Autodesk Fusion 360 part; units mm, degrees
note: some values were not read from the file. Chosen so that the rebuilt part matches the saved one: which bodies a step acts on.
(part 2 of 3)
  line L404 (275.1852, -92.964) -> (274.8216, -92.964)
  line L405 (274.8216, -92.964) -> (274.8216, -90.0604)
  arc A366 (268.6669, -89.5604) -> (268.1669, -90.0604) centre (268.6669, -90.0604) ccw
  arc A367 (268.1669, -101.5666) -> (267.6669, -101.0666) centre (267.6669, -101.5666) ccw
  arc A368 (269.9703, -102.354) -> (269.4703, -101.854) centre (269.4703, -102.354) ccw
  arc A369 (269.9703, -102.5224) -> (270.4703, -103.0224) centre (270.4703, -102.5224) ccw
  arc A370 (272.5183, -103.0224) -> (273.0183, -102.5224) centre (272.5183, -102.5224) ccw
  arc A371 (273.5183, -101.854) -> (273.0183, -102.354) centre (273.5183, -102.354) ccw
  arc A372 (274.3216, -101.854) -> (274.8216, -101.354) centre (274.3216, -101.354) ccw
  arc A373 (275.3216, -95.758) -> (274.8216, -96.258) centre (275.3216, -96.258) ccw
  arc A374 (275.6852, -93.464) -> (275.1852, -92.964) centre (275.1852, -93.464) ccw
  arc A375 (274.8216, -90.0604) -> (274.3216, -89.5604) centre (274.3216, -90.0604) ccw
  line L406 (293.5375, -88.25) -> (306.5375, -88.25)
  line L407 (293.5375, -102.25) -> (306.5375, -102.25)
  line L408 (293.0375, -88.75) -> (293.0375, -101.75)
  line L409 (307.0375, -88.75) -> (307.0375, -101.75)
  arc A376 (293.5375, -88.25) -> (293.0375, -88.75) centre (293.5375, -88.75) ccw
  arc A377 (307.0375, -88.75) -> (306.5375, -88.25) centre (306.5375, -88.75) ccw
  arc A378 (293.0375, -101.75) -> (293.5375, -102.25) centre (293.5375, -101.75) ccw
  arc A379 (306.5375, -102.25) -> (307.0375, -101.75) centre (306.5375, -101.75) ccw
  line L410 (312.5875, -88.25) -> (325.5875, -88.25)
  line L411 (312.5875, -102.25) -> (325.5875, -102.25)
  line L412 (312.0875, -88.75) -> (312.0875, -101.75)
  line L413 (326.0875, -88.75) -> (326.0875, -101.75)
  arc A380 (312.5875, -88.25) -> (312.0875, -88.75) centre (312.5875, -88.75) ccw
  arc A381 (326.0875, -88.75) -> (325.5875, -88.25) centre (325.5875, -88.75) ccw
  arc A382 (312.0875, -101.75) -> (312.5875, -102.25) centre (312.5875, -101.75) ccw
  arc A383 (325.5875, -102.25) -> (326.0875, -101.75) centre (325.5875, -101.75) ccw
  line L414 (331.6375, -88.25) -> (344.6375, -88.25)
  line L415 (331.6375, -102.25) -> (344.6375, -102.25)
  line L416 (331.1375, -88.75) -> (331.1375, -101.75)
  line L417 (345.1375, -88.75) -> (345.1375, -101.75)
  arc A384 (331.6375, -88.25) -> (331.1375, -88.75) centre (331.6375, -88.75) ccw
  arc A385 (345.1375, -88.75) -> (344.6375, -88.25) centre (344.6375, -88.75) ccw
  arc A386 (331.1375, -101.75) -> (331.6375, -102.25) centre (331.6375, -101.75) ccw
  arc A387 (344.6375, -102.25) -> (345.1375, -101.75) centre (344.6375, -101.75) ccw
  line L418 (5.4062, -107.3) -> (18.4063, -107.3)
  line L419 (5.4062, -121.3) -> (18.4063, -121.3)
  line L420 (4.9062, -107.8) -> (4.9062, -120.8)
  line L421 (18.9062, -107.8) -> (18.9062, -120.8)
  arc A388 (5.4062, -107.3) -> (4.9062, -107.8) centre (5.4062, -107.8) ccw
  arc A389 (18.9062, -107.8) -> (18.4062, -107.3) centre (18.4062, -107.8) ccw
  arc A390 (4.9062, -120.8) -> (5.4062, -121.3) centre (5.4062, -120.8) ccw
  arc A391 (18.4062, -121.3) -> (18.9063, -120.8) centre (18.4062, -120.8) ccw
  line L422 (29.2188, -107.3) -> (42.2188, -107.3)
  line L423 (29.2188, -121.3) -> (42.2188, -121.3)
  line L424 (28.7188, -107.8) -> (28.7188, -120.8)
  line L425 (42.7188, -107.8) -> (42.7188, -120.8)
  arc A392 (29.2188, -107.3) -> (28.7187, -107.8) centre (29.2188, -107.8) ccw
  arc A393 (42.7188, -107.8) -> (42.2188, -107.3) centre (42.2188, -107.8) ccw
  arc A394 (28.7188, -120.8) -> (29.2188, -121.3) centre (29.2188, -120.8) ccw
  arc A395 (42.2188, -121.3) -> (42.7188, -120.8) centre (42.2188, -120.8) ccw
  line L426 (53.0313, -107.3) -> (66.0312, -107.3)
  line L427 (53.0313, -121.3) -> (66.0312, -121.3)
  line L428 (52.5313, -107.8) -> (52.5313, -120.8)
  line L429 (66.5312, -107.8) -> (66.5312, -120.8)
  arc A396 (53.0313, -107.3) -> (52.5312, -107.8) centre (53.0313, -107.8) ccw
  arc A397 (66.5312, -107.8) -> (66.0312, -107.3) centre (66.0312, -107.8) ccw
  arc A398 (52.5313, -120.8) -> (53.0313, -121.3) centre (53.0313, -120.8) ccw
  arc A399 (66.0312, -121.3) -> (66.5312, -120.8) centre (66.0312, -120.8) ccw
  line L430 (124.4688, -107.3) -> (137.4688, -107.3)
  line L431 (124.4688, -121.3) -> (137.4688, -121.3)
  line L432 (123.9688, -107.8) -> (123.9688, -120.8)
  line L433 (137.9688, -107.8) -> (137.9688, -120.8)
  arc A400 (124.4688, -107.3) -> (123.9688, -107.8) centre (124.4688, -107.8) ccw
  arc A401 (137.9688, -107.8) -> (137.4688, -107.3) centre (137.4688, -107.8) ccw
  arc A402 (123.9688, -120.8) -> (124.4688, -121.3) centre (124.4688, -120.8) ccw
  arc A403 (137.4688, -121.3) -> (137.9688, -120.8) centre (137.4688, -120.8) ccw
  line L434 (78.1414, -108.6104) -> (83.7961, -108.6104)
  line L435 (84.2961, -109.1104) -> (84.2961, -111.5)
  line L436 (84.7962, -112) -> (130.9688, -112)
  line L437 (130.9688, -116.6) -> (84.7961, -116.6)
  line L438 (84.2961, -117.1) -> (84.2961, -120.404)
  line L439 (83.7961, -120.904) -> (82.9928, -120.904)
  line L440 (82.4928, -121.404) -> (82.4928, -121.5724)
  line L441 (81.9928, -122.0724) -> (79.9447, -122.0724)
  line L442 (79.4447, -121.5724) -> (79.4447, -121.404)
  line L443 (78.9447, -120.904) -> (78.1414, -120.904)
  line L444 (77.6414, -120.404) -> (77.6414, -115.308)
  line L445 (77.1414, -114.808) -> (76.7777, -114.808)
  line L446 (76.7777, -114.808) -> (76.7777, -112.514)
  line L447 (77.2777, -112.014) -> (77.6414, -112.014)
  line L448 (77.6414, -112.014) -> (77.6414, -109.1104)
  arc A404 (84.2962, -109.1104) -> (83.7961, -108.6104) centre (83.7961, -109.1104) ccw
  arc A405 (84.2962, -111.5) -> (84.7962, -112) centre (84.7962, -111.5) ccw
  arc A406 (84.7962, -116.6) -> (84.2962, -117.1) centre (84.7962, -117.1) ccw
  arc A407 (83.7961, -120.904) -> (84.2962, -120.404) centre (83.7961, -120.404) ccw
  arc A408 (82.9928, -120.904) -> (82.4928, -121.404) centre (82.9928, -121.404) ccw
  arc A409 (81.9928, -122.0724) -> (82.4927, -121.5724) centre (81.9928, -121.5724) ccw
  arc A410 (79.4447, -121.5724) -> (79.9447, -122.0724) centre (79.9447, -121.5724) ccw
  arc A411 (79.4447, -121.404) -> (78.9447, -120.904) centre (78.9447, -121.404) ccw
  arc A412 (77.6414, -120.404) -> (78.1414, -120.904) centre (78.1414, -120.404) ccw
  arc A413 (77.6414, -115.308) -> (77.1414, -114.808) centre (77.1414, -115.308) ccw
  arc A414 (77.2777, -112.014) -> (76.7777, -112.514) centre (77.2777, -112.514) ccw
  arc A415 (78.1414, -108.6104) -> (77.6414, -109.1104) centre (78.1414, -109.1104) ccw
  line L449 (183.7962, -108.6104) -> (178.1413, -108.6104)
  line L450 (177.6413, -109.1104) -> (177.6413, -111.5)
  line L451 (177.1413, -112) -> (130.9688, -112)
  line L452 (130.9688, -116.6) -> (177.1413, -116.6)
  line L453 (177.6413, -117.1) -> (177.6413, -120.404)
  line L454 (178.1413, -120.904) -> (178.9447, -120.904)
  line L455 (179.4447, -121.404) -> (179.4447, -121.5724)
  line L456 (179.9447, -122.0724) -> (181.9928, -122.0724)
  line L457 (182.4928, -121.5724) -> (182.4928, -121.404)
  line L458 (182.9928, -120.904) -> (183.7962, -120.904)
  line L459 (184.2962, -120.404) -> (184.2962, -115.308)
  line L460 (184.7962, -114.808) -> (185.1598, -114.808)
  line L461 (185.1598, -114.808) -> (185.1598, -112.514)
  line L462 (184.6598, -112.014) -> (184.2962, -112.014)
  line L463 (184.2962, -112.014) -> (184.2962, -109.1104)
  arc A416 (178.1413, -108.6104) -> (177.6413, -109.1104) centre (178.1413, -109.1104) ccw
  arc A417 (177.1413, -112) -> (177.6413, -111.5) centre (177.1413, -111.5) ccw
  arc A418 (177.6413, -117.1) -> (177.1413, -116.6) centre (177.1413, -117.1) ccw
  arc A419 (177.6413, -120.404) -> (178.1413, -120.904) centre (178.1413, -120.404) ccw
  arc A420 (179.4447, -121.404) -> (178.9447, -120.904) centre (178.9447, -121.404) ccw
  arc A421 (179.4447, -121.5724) -> (179.9447, -122.0724) centre (179.9447, -121.5724) ccw
  arc A422 (181.9928, -122.0724) -> (182.4928, -121.5724) centre (181.9928, -121.5724) ccw
  arc A423 (182.9928, -120.904) -> (182.4928, -121.404) centre (182.9928, -121.404) ccw
  arc A424 (183.7962, -120.904) -> (184.2962, -120.404) centre (183.7962, -120.404) ccw
  arc A425 (184.7962, -114.808) -> (184.2962, -115.308) centre (184.7962, -115.308) ccw
  arc A426 (185.1598, -112.514) -> (184.6598, -112.014) centre (184.6598, -112.514) ccw
  arc A427 (184.2962, -109.1104) -> (183.7962, -108.6104) centre (183.7962, -109.1104) ccw
  line L464 (195.9063, -107.3) -> (208.9062, -107.3)
  line L465 (195.9063, -121.3) -> (208.9062, -121.3)
  line L466 (195.4063, -107.8) -> (195.4063, -120.8)
  line L467 (209.4062, -107.8) -> (209.4062, -120.8)
  arc A428 (195.9063, -107.3) -> (195.4063, -107.8) centre (195.9063, -107.8) ccw
  arc A429 (209.4062, -107.8) -> (208.9062, -107.3) centre (208.9062, -107.8) ccw
  arc A430 (195.4063, -120.8) -> (195.9063, -121.3) centre (195.9063, -120.8) ccw
  arc A431 (208.9062, -121.3) -> (209.4062, -120.8) centre (208.9062, -120.8) ccw
  line L468 (219.7188, -107.3) -> (232.7188, -107.3)
  line L469 (219.7188, -121.3) -> (232.7188, -121.3)
  line L470 (219.2188, -107.8) -> (219.2188, -120.8)
  line L471 (233.2188, -107.8) -> (233.2188, -120.8)
  arc A432 (219.7188, -107.3) -> (219.2188, -107.8) centre (219.7188, -107.8) ccw
  arc A433 (233.2188, -107.8) -> (232.7188, -107.3) centre (232.7188, -107.8) ccw
  arc A434 (219.2188, -120.8) -> (219.7188, -121.3) centre (219.7188, -120.8) ccw
  arc A435 (232.7188, -121.3) -> (233.2188, -120.8) centre (232.7188, -120.8) ccw
  line L472 (243.5313, -107.3) -> (256.5313, -107.3)
  line L473 (243.5313, -121.3) -> (256.5313, -121.3)
  line L474 (243.0312, -107.8) -> (243.0312, -120.8)
  line L475 (257.0312, -107.8) -> (257.0312, -120.8)
  arc A436 (243.5313, -107.3) -> (243.0313, -107.8) centre (243.5313, -107.8) ccw
  arc A437 (257.0312, -107.8) -> (256.5312, -107.3) centre (256.5312, -107.8) ccw
  arc A438 (243.0313, -120.8) -> (243.5313, -121.3) centre (243.5313, -120.8) ccw
  arc A439 (256.5312, -121.3) -> (257.0312, -120.8) centre (256.5312, -120.8) ccw
  line L476 (267.3438, -107.3) -> (280.3438, -107.3)
  line L477 (267.3438, -121.3) -> (280.3438, -121.3)
  line L478 (266.8438, -107.8) -> (266.8438, -120.8)
  line L479 (280.8438, -107.8) -> (280.8438, -120.8)
  arc A440 (267.3438, -107.3) -> (266.8438, -107.8) centre (267.3438, -107.8) ccw
  arc A441 (280.8438, -107.8) -> (280.3438, -107.3) centre (280.3438, -107.8) ccw
  arc A442 (266.8438, -120.8) -> (267.3438, -121.3) centre (267.3438, -120.8) ccw
  arc A443 (280.3438, -121.3) -> (280.8438, -120.8) centre (280.3438, -120.8) ccw
  line L480 (293.5375, -107.3) -> (306.5375, -107.3)
  line L481 (293.5375, -121.3) -> (306.5375, -121.3)
  line L482 (293.0375, -107.8) -> (293.0375, -120.8)
  line L483 (307.0375, -107.8) -> (307.0375, -120.8)
  arc A444 (293.5375, -107.3) -> (293.0375, -107.8) centre (293.5375, -107.8) ccw
  arc A445 (307.0375, -107.8) -> (306.5375, -107.3) centre (306.5375, -107.8) ccw
  arc A446 (293.0375, -120.8) -> (293.5375, -121.3) centre (293.5375, -120.8) ccw
  arc A447 (306.5375, -121.3) -> (307.0375, -120.8) centre (306.5375, -120.8) ccw
  line L484 (312.5875, -107.3) -> (325.5875, -107.3)
  line L485 (312.5875, -121.3) -> (325.5875, -121.3)
  line L486 (312.0875, -107.8) -> (312.0875, -120.8)
  line L487 (326.0875, -107.8) -> (326.0875, -120.8)
  arc A448 (312.5875, -107.3) -> (312.0875, -107.8) centre (312.5875, -107.8) ccw
  arc A449 (326.0875, -107.8) -> (325.5875, -107.3) centre (325.5875, -107.8) ccw
  arc A450 (312.0875, -120.8) -> (312.5875, -121.3) centre (312.5875, -120.8) ccw
  arc A451 (325.5875, -121.3) -> (326.0875, -120.8) centre (325.5875, -120.8) ccw
  line L488 (331.6375, -107.3) -> (344.6375, -107.3)
  line L489 (331.6375, -121.3) -> (344.6375, -121.3)
  line L490 (331.1375, -107.8) -> (331.1375, -120.8)
  line L491 (345.1375, -107.8) -> (345.1375, -120.8)
  arc A452 (331.6375, -107.3) -> (331.1375, -107.8) centre (331.6375, -107.8) ccw
  arc A453 (345.1375, -107.8) -> (344.6375, -107.3) centre (344.6375, -107.8) ccw
  arc A454 (331.1375, -120.8) -> (331.6375, -121.3) centre (331.6375, -120.8) ccw
  arc A455 (344.6375, -121.3) -> (345.1375, -120.8) centre (344.6375, -120.8) ccw
  line L492 (0, -123.825) -> (347.6625, -123.825)
  line L493 (0, 0) -> (347.6625, 0)
  line L494 (0, -123.825) -> (0, 0)
  line L495 (347.6625, -123.825) -> (347.6625, 0)
extrude "Extrude1" add sketch "plate-2026-02-23T17_51_34.543Z" along normal blind 1.5 makes body 1
extrude "Extrude2" add 1 faces at (0, 0.5, 82.55) along direction (-1, 0, 0) blind 2 on bodies 1 bodies 1
extrude "Extrude3" add 1 faces at (114.5542, 1, 123.825) along direction (0, 0, 1) blind 4 on bodies 1 bodies 1
extrude "Extrude4" add 1 faces at (347.6625, 0.5, 42.6083) along direction (1, 0, 0) blind 31.5 on bodies 1 bodies 1
extrude "Extrude5" add 1 faces at (252.1083, 1, 0) along direction (0, 0, -1) blind 3 on bodies 1 bodies 1
extrude "Extrude6" add 1 faces at (125.0542, 0.5, 127.825) along direction (0, 0, 1) blind 1 on bodies 1 bodies 1
sketch "Sketch2" plane through (0, 1.5, 0) normal (0, 1, 0) x (-1, 0, 0)
  arc A0 (-312.5875, 88.25) -> (-312.0875, 88.75) centre (-312.5875, 88.75) ccw
  line L0 (-312.5875, 88.25) -> (-325.5875, 88.25)
  arc A1 (-326.0875, 88.75) -> (-325.5875, 88.25) centre (-325.5875, 88.75) ccw
  line L1 (-326.0875, 88.75) -> (-326.0875, 101.75)
  arc A2 (-325.5875, 102.25) -> (-326.0875, 101.75) centre (-325.5875, 101.75) ccw
  line L2 (-325.5875, 102.25) -> (-312.5875, 102.25)
  arc A3 (-312.0875, 101.75) -> (-312.5875, 102.25) centre (-312.5875, 101.75) ccw
  line L3 (-312.0875, 101.75) -> (-312.0875, 88.75)
  arc A4 (-331.6375, 88.25) -> (-331.1375, 88.75) centre (-331.6375, 88.75) ccw
  line L4 (-331.6375, 88.25) -> (-344.6375, 88.25)
  arc A5 (-345.1375, 88.75) -> (-344.6375, 88.25) centre (-344.6375, 88.75) ccw
  line L5 (-345.1375, 88.75) -> (-345.1375, 101.75)
  arc A6 (-344.6375, 102.25) -> (-345.1375, 101.75) centre (-344.6375, 101.75) ccw
  line L6 (-344.6375, 102.25) -> (-331.6375, 102.25)
  arc A7 (-331.1375, 101.75) -> (-331.6375, 102.25) centre (-331.6375, 101.75) ccw
  line L7 (-331.1375, 101.75) -> (-331.1375, 88.75)
  arc A8 (-53.0313, 107.3) -> (-52.5312, 107.8) centre (-53.0313, 107.8) ccw
  line L8 (-53.0313, 107.3) -> (-66.0312, 107.3)
  arc A9 (-66.5312, 107.8) -> (-66.0312, 107.3) centre (-66.0312, 107.8) ccw
  line L9 (-66.5312, 107.8) -> (-66.5313, 120.8)
  arc A10 (-66.0313, 121.3) -> (-66.5313, 120.8) centre (-66.0312, 120.8) ccw
  line L10 (-66.0312, 121.3) -> (-53.0313, 121.3)
  arc A11 (-52.5313, 120.8) -> (-53.0313, 121.3) centre (-53.0312, 120.8) ccw
  line L11 (-52.5313, 120.8) -> (-52.5312, 107.8)
  line L12 (-185.1598, 114.808) -> (-184.7962, 114.808)
  arc A12 (-184.7962, 114.808) -> (-184.2962, 115.308) centre (-184.7962, 115.308) ccw
  line L13 (-184.2962, 115.308) -> (-184.2962, 120.404)
  arc A13 (-183.7962, 120.904) -> (-184.2962, 120.404) centre (-183.7962, 120.404) ccw
  line L14 (-183.7962, 120.904) -> (-182.9928, 120.904)
  arc A14 (-182.9928, 120.904) -> (-182.4928, 121.404) centre (-182.9928, 121.404) ccw
  line L15 (-182.4928, 121.404) -> (-182.4928, 121.5724)
  arc A15 (-181.9928, 122.0724) -> (-182.4927, 121.5724) centre (-181.9927, 121.5724) ccw
  line L16 (-181.9928, 122.0724) -> (-179.9447, 122.0724)
  arc A16 (-179.4447, 121.5724) -> (-179.9447, 122.0724) centre (-179.9447, 121.5724) ccw
  line L17 (-179.4447, 121.5724) -> (-179.4447, 121.404)
  arc A17 (-179.4447, 121.404) -> (-178.9447, 120.904) centre (-178.9447, 121.404) ccw
  line L18 (-178.9447, 120.904) -> (-178.1413, 120.904)
  arc A18 (-177.6413, 120.404) -> (-178.1413, 120.904) centre (-178.1413, 120.404) ccw
  line L19 (-177.6413, 120.404) -> (-177.6413, 117.1)
  arc A19 (-177.6413, 117.1) -> (-177.1413, 116.6) centre (-177.1413, 117.1) ccw
  line L20 (-177.1413, 116.6) -> (-137.9688, 116.6)
  line L21 (-137.9688, 116.6) -> (-137.9688, 120.8)
  arc A20 (-137.4688, 121.3) -> (-137.9688, 120.8) centre (-137.4687, 120.8) ccw
  line L22 (-137.4688, 121.3) -> (-124.4687, 121.3)
  arc A21 (-123.9688, 120.8) -> (-124.4687, 121.3) centre (-124.4688, 120.8) ccw
  line L23 (-123.9688, 120.8) -> (-123.9688, 116.6)
  line L24 (-123.9688, 116.6) -> (-84.7962, 116.6)
  arc A22 (-84.7962, 116.6) -> (-84.2962, 117.1) centre (-84.7962, 117.1) ccw
  line L25 (-84.2961, 117.1) -> (-84.2961, 120.404)
  arc A23 (-83.7961, 120.904) -> (-84.2961, 120.404) centre (-83.7961, 120.404) ccw
  line L26 (-83.7961, 120.904) -> (-82.9928, 120.904)
  arc A24 (-82.9928, 120.904) -> (-82.4928, 121.404) centre (-82.9928, 121.404) ccw
  line L27 (-82.4928, 121.404) -> (-82.4927, 121.5724)
  arc A25 (-81.9928, 122.0724) -> (-82.4927, 121.5724) centre (-81.9928, 121.5724) ccw
  line L28 (-81.9928, 122.0724) -> (-79.9448, 122.0724)
  arc A26 (-79.4447, 121.5724) -> (-79.9448, 122.0724) centre (-79.9448, 121.5724) ccw
  line L29 (-79.4447, 121.5724) -> (-79.4447, 121.404)
  arc A27 (-79.4447, 121.404) -> (-78.9447, 120.904) centre (-78.9447, 121.404) ccw
  line L30 (-78.9447, 120.904) -> (-78.1414, 120.904)
  arc A28 (-77.6414, 120.404) -> (-78.1414, 120.904) centre (-78.1413, 120.404) ccw
  line L31 (-77.6414, 120.404) -> (-77.6413, 115.308)
  arc A29 (-77.6413, 115.308) -> (-77.1414, 114.808) centre (-77.1414, 115.308) ccw
  line L32 (-77.1414, 114.808) -> (-76.7777, 114.808)
  line L33 (-76.7777, 114.808) -> (-76.7777, 112.514)
  arc A30 (-77.2777, 112.014) -> (-76.7777, 112.514) centre (-77.2777, 112.514) ccw
  line L34 (-77.2777, 112.014) -> (-77.6413, 112.014)
  line L35 (-77.6413, 112.014) -> (-77.6414, 109.1104)
  arc A31 (-78.1414, 108.6104) -> (-77.6414, 109.1104) centre (-78.1413, 109.1104) ccw
  line L36 (-78.1414, 108.6104) -> (-83.7962, 108.6104)
  arc A32 (-84.2962, 109.1104) -> (-83.7962, 108.6104) centre (-83.7961, 109.1104) ccw
  line L37 (-84.2961, 109.1104) -> (-84.2961, 111.5)
  arc A33 (-84.2961, 111.5) -> (-84.7962, 112) centre (-84.7962, 111.5) ccw
  line L38 (-84.7962, 112) -> (-123.9688, 112)
  line L39 (-123.9688, 112) -> (-123.9688, 107.8)
  arc A34 (-124.4688, 107.3) -> (-123.9688, 107.8) centre (-124.4688, 107.8) ccw
  line L40 (-124.4688, 107.3) -> (-137.4688, 107.3)
  arc A35 (-137.9688, 107.8) -> (-137.4688, 107.3) centre (-137.4688, 107.8) ccw
  line L41 (-137.9688, 107.8) -> (-137.9688, 112)
  line L42 (-137.9688, 112) -> (-177.1413, 112)
  arc A36 (-177.1413, 112) -> (-177.6413, 111.5) centre (-177.1413, 111.5) ccw
  line L43 (-177.6413, 111.5) -> (-177.6414, 109.1104)
  arc A37 (-178.1414, 108.6104) -> (-177.6414, 109.1104) centre (-178.1414, 109.1104) ccw
  line L44 (-178.1413, 108.6104) -> (-183.7962, 108.6104)
  arc A38 (-184.2962, 109.1104) -> (-183.7962, 108.6104) centre (-183.7962, 109.1104) ccw
  line L45 (-184.2962, 109.1104) -> (-184.2962, 112.014)
  line L46 (-184.2962, 112.014) -> (-184.6598, 112.014)
  arc A39 (-185.1598, 112.514) -> (-184.6598, 112.014) centre (-184.6598, 112.514) ccw
  line L47 (-185.1598, 112.514) -> (-185.1598, 114.808)
  arc A40 (-250.675, 2.525) -> (-250.175, 3.025) centre (-250.675, 3.025) ccw
  line L48 (-250.675, 2.525) -> (-263.675, 2.525)
  arc A41 (-264.175, 3.025) -> (-263.675, 2.525) centre (-263.675, 3.025) ccw
  line L49 (-264.175, 3.025) -> (-264.175, 16.025)
  arc A42 (-263.675, 16.525) -> (-264.175, 16.025) centre (-263.675, 16.025) ccw
  line L50 (-263.675, 16.525) -> (-250.675, 16.525)
  arc A43 (-250.175, 16.025) -> (-250.675, 16.525) centre (-250.675, 16.025) ccw
  line L51 (-250.175, 16.025) -> (-250.175, 3.025)
  arc A44 (-312.5875, 69.2) -> (-312.0875, 69.7) centre (-312.5875, 69.7) ccw
  line L52 (-312.5875, 69.2) -> (-325.5875, 69.2)
  arc A45 (-326.0875, 69.7) -> (-325.5875, 69.2) centre (-325.5875, 69.7) ccw
  line L53 (-326.0875, 69.7) -> (-326.0875, 82.7)
  arc A46 (-325.5875, 83.2) -> (-326.0875, 82.7) centre (-325.5875, 82.7) ccw
  line L54 (-325.5875, 83.2) -> (-312.5875, 83.2)
  arc A47 (-312.0875, 82.7) -> (-312.5875, 83.2) centre (-312.5875, 82.7) ccw
  line L55 (-312.0875, 82.7) -> (-312.0875, 69.7)
  arc A48 (-160.1875, 88.25) -> (-159.6875, 88.75) centre (-160.1875, 88.75) ccw
  line L56 (-160.1875, 88.25) -> (-173.1875, 88.25)
  arc A49 (-173.6875, 88.75) -> (-173.1875, 88.25) centre (-173.1875, 88.75) ccw
  line L57 (-173.6875, 88.75) -> (-173.6875, 101.75)
  arc A50 (-173.1875, 102.25) -> (-173.6875, 101.75) centre (-173.1875, 101.75) ccw
  line L58 (-173.1875, 102.25) -> (-160.1875, 102.25)
  arc A51 (-159.6875, 101.75) -> (-160.1875, 102.25) centre (-160.1875, 101.75) ccw
  line L59 (-159.6875, 101.75) -> (-159.6875, 88.75)
  arc A52 (-117.325, 31.1) -> (-116.825, 31.6) centre (-117.325, 31.6) ccw
  line L60 (-117.325, 31.1) -> (-130.325, 31.1)
  arc A53 (-130.825, 31.6) -> (-130.325, 31.1) centre (-130.325, 31.6) ccw
  line L61 (-130.825, 31.6) -> (-130.825, 44.6)
  arc A54 (-130.325, 45.1) -> (-130.825, 44.6) centre (-130.325, 44.6) ccw
  line L62 (-130.325, 45.1) -> (-117.325, 45.1)
  arc A55 (-116.825, 44.6) -> (-117.325, 45.1) centre (-117.325, 44.6) ccw
  line L63 (-116.825, 44.6) -> (-116.825, 31.6)
  arc A56 (-98.275, 31.1) -> (-97.775, 31.6) centre (-98.275, 31.6) ccw
  line L64 (-98.275, 31.1) -> (-111.275, 31.1)
  arc A57 (-111.775, 31.6) -> (-111.275, 31.1) centre (-111.275, 31.6) ccw
  line L65 (-111.775, 31.6) -> (-111.775, 44.6)
  arc A58 (-111.275, 45.1) -> (-111.775, 44.6) centre (-111.275, 44.6) ccw
  line L66 (-111.275, 45.1) -> (-98.275, 45.1)
  arc A59 (-97.775, 44.6) -> (-98.275, 45.1) centre (-98.275, 44.6) ccw
  line L67 (-97.775, 44.6) -> (-97.775, 31.6)
  arc A60 (-245.9125, 69.2) -> (-245.4125, 69.7) centre (-245.9125, 69.7) ccw
  line L68 (-245.9125, 69.2) -> (-258.9125, 69.2)
  arc A61 (-259.4125, 69.7) -> (-258.9125, 69.2) centre (-258.9125, 69.7) ccw
  line L69 (-259.4125, 69.7) -> (-259.4125, 82.7)
  arc A62 (-258.9125, 83.2) -> (-259.4125, 82.7) centre (-258.9125, 82.7) ccw
  line L70 (-258.9125, 83.2) -> (-245.9125, 83.2)
  arc A63 (-245.4125, 82.7) -> (-245.9125, 83.2) centre (-245.9125, 82.7) ccw
  line L71 (-245.4125, 82.7) -> (-245.4125, 69.7)
  line L72 (-273.3358, 82.804) -> (-273.3358, 82.4404)
  arc A64 (-273.3358, 82.4404) -> (-272.8358, 81.9404) centre (-272.8358, 82.4404) ccw
  line L73 (-272.8358, 81.9404) -> (-267.7398, 81.9404)
  arc A65 (-267.2398, 81.4404) -> (-267.7398, 81.9404) centre (-267.7398, 81.4404) ccw
  line L74 (-267.2398, 81.4404) -> (-267.2398, 80.637)
  arc A66 (-267.2398, 80.637) -> (-266.7398, 80.137) centre (-266.7398, 80.637) ccw
  line L75 (-266.7398, 80.137) -> (-266.5713, 80.137)
  arc A67 (-266.0713, 79.637) -> (-266.5713, 80.137) centre (-266.5713, 79.637) ccw
  line L76 (-266.0713, 79.637) -> (-266.0713, 77.589)
  arc A68 (-266.5713, 77.089) -> (-266.0713, 77.589) centre (-266.5713, 77.589) ccw
  line L77 (-266.5713, 77.089) -> (-266.7398, 77.089)
  arc A69 (-266.7398, 77.089) -> (-267.2398, 76.589) centre (-266.7398, 76.589) ccw
  line L78 (-267.2398, 76.589) -> (-267.2398, 75.2856)
  line L79 (-267.2398, 75.2856) -> (-267.5272, 75.2856)
  arc A70 (-267.5272, 75.2856) -> (-268.0272, 74.7856) centre (-267.5272, 74.7856) ccw
  line L80 (-268.0272, 74.7856) -> (-268.0272, 73.675)
  line L81 (-268.0272, 73.675) -> (-267.3438, 73.675)
  arc A71 (-266.8438, 73.175) -> (-267.3438, 73.675) centre (-267.3438, 73.175) ccw
  line L82 (-266.8438, 73.175) -> (-266.8437, 60.175)
  arc A72 (-267.3438, 59.675) -> (-266.8438, 60.175) centre (-267.3438, 60.175) ccw
  line L83 (-267.3438, 59.675) -> (-268.0272, 59.675)
  line L84 (-268.0272, 59.675) -> (-268.0272, 58.5644)
  arc A73 (-268.0272, 58.5644) -> (-267.5272, 58.0644) centre (-267.5272, 58.5644) ccw
  line L85 (-267.5272, 58.0644) -> (-267.2398, 58.0644)
  line L86 (-267.2398, 58.0644) -> (-267.2398, 56.761)
  arc A74 (-267.2398, 56.761) -> (-266.7398, 56.261) centre (-266.7398, 56.761) ccw
  line L87 (-266.7398, 56.261) -> (-266.5713, 56.261)
  arc A75 (-266.0713, 55.761) -> (-266.5713, 56.261) centre (-266.5713, 55.761) ccw
  line L88 (-266.0713, 55.761) -> (-266.0713, 53.713)
  arc A76 (-266.5713, 53.213) -> (-266.0713, 53.713) centre (-266.5713, 53.713) ccw
  line L89 (-266.5713, 53.213) -> (-266.7398, 53.213)
  arc A77 (-266.7398, 53.213) -> (-267.2398, 52.713) centre (-266.7398, 52.713) ccw
  line L90 (-267.2398, 52.713) -> (-267.2398, 51.9096)
  arc A78 (-267.7398, 51.4096) -> (-267.2398, 51.9096) centre (-267.7398, 51.9096) ccw
  line L91 (-267.7398, 51.4096) -> (-272.8358, 51.4096)
  arc A79 (-272.8358, 51.4096) -> (-273.3358, 50.9096) centre (-272.8358, 50.9096) ccw
  line L92 (-273.3358, 50.9096) -> (-273.3358, 50.546)
  line L93 (-273.3358, 50.546) -> (-275.6298, 50.546)
  arc A80 (-276.1298, 51.046) -> (-275.6298, 50.546) centre (-275.6298, 51.046) ccw
  line L94 (-276.1298, 51.046) -> (-276.1298, 51.4096)
  line L95 (-276.1298, 51.4096) -> (-279.0333, 51.4096)
  arc A81 (-279.5334, 51.9096) -> (-279.0333, 51.4096) centre (-279.0334, 51.9096) ccw
  line L96 (-279.5333, 51.9096) -> (-279.5333, 57.5644)
  arc A82 (-279.0333, 58.0644) -> (-279.5333, 57.5644) centre (-279.0333, 57.5644) ccw
  line L97 (-279.0333, 58.0644) -> (-278.7206, 58.0644)
  line L98 (-278.7206, 58.0644) -> (-278.7206, 59.675)
  line L99 (-278.7206, 59.675) -> (-280.3438, 59.675)
  arc A83 (-280.8438, 60.175) -> (-280.3438, 59.675) centre (-280.3438, 60.175) ccw
  line L100 (-280.8438, 60.175) -> (-280.8438, 73.175)
  arc A84 (-280.3438, 73.675) -> (-280.8438, 73.175) centre (-280.3438, 73.175) ccw
  line L101 (-280.3438, 73.675) -> (-278.7206, 73.675)
  line L102 (-278.7206, 73.675) -> (-278.7206, 75.2856)
  line L103 (-278.7206, 75.2856) -> (-279.0333, 75.2856)
  arc A85 (-279.5334, 75.7856) -> (-279.0333, 75.2856) centre (-279.0334, 75.7856) ccw
  line L104 (-279.5333, 75.7856) -> (-279.5333, 81.4404)
  arc A86 (-279.0333, 81.9404) -> (-279.5333, 81.4404) centre (-279.0333, 81.4404) ccw
  line L105 (-279.0333, 81.9404) -> (-276.1298, 81.9404)
  line L106 (-276.1298, 81.9404) -> (-276.1297, 82.304)
  arc A87 (-275.6298, 82.804) -> (-276.1298, 82.304) centre (-275.6298, 82.304) ccw
  line L107 (-275.6298, 82.804) -> (-273.3358, 82.804)
  arc A88 (-219.7188, 107.3) -> (-219.2188, 107.8) centre (-219.7187, 107.8) ccw
  line L108 (-219.7188, 107.3) -> (-232.7188, 107.3)
  arc A89 (-233.2188, 107.8) -> (-232.7188, 107.3) centre (-232.7188, 107.8) ccw
  line L109 (-233.2188, 107.8) -> (-233.2188, 120.8)
  arc A90 (-232.7188, 121.3) -> (-233.2188, 120.8) centre (-232.7188, 120.8) ccw
  line L110 (-232.7188, 121.3) -> (-219.7188, 121.3)
  arc A91 (-219.2188, 120.8) -> (-219.7188, 121.3) centre (-219.7188, 120.8) ccw
  line L111 (-219.2188, 120.8) -> (-219.2188, 107.8)
  arc A92 (-103.0375, 88.25) -> (-102.5375, 88.75) centre (-103.0375, 88.75) ccw
  line L112 (-103.0375, 88.25) -> (-116.0375, 88.25)
  arc A93 (-116.5375, 88.75) -> (-116.0375, 88.25) centre (-116.0375, 88.75) ccw
  line L113 (-116.5375, 88.75) -> (-116.5375, 101.75)
  arc A94 (-116.0375, 102.25) -> (-116.5375, 101.75) centre (-116.0375, 101.75) ccw
  line L114 (-116.0375, 102.25) -> (-103.0375, 102.25)
  arc A95 (-102.5375, 101.75) -> (-103.0375, 102.25) centre (-103.0375, 101.75) ccw
  line L115 (-102.5375, 101.75) -> (-102.5375, 88.75)
  arc A96 (-267.3438, 107.3) -> (-266.8438, 107.8) centre (-267.3438, 107.8) ccw
  line L116 (-267.3438, 107.3) -> (-280.3438, 107.3)
  arc A97 (-280.8438, 107.8) -> (-280.3438, 107.3) centre (-280.3438, 107.8) ccw
  line L117 (-280.8438, 107.8) -> (-280.8438, 120.8)
  arc A98 (-280.3438, 121.3) -> (-280.8438, 120.8) centre (-280.3438, 120.8) ccw
  line L118 (-280.3438, 121.3) -> (-267.3438, 121.3)
  arc A99 (-266.8438, 120.8) -> (-267.3438, 121.3) centre (-267.3438, 120.8) ccw
  line L119 (-266.8438, 120.8) -> (-266.8438, 107.8)
  arc A100 (-293.5375, 107.3) -> (-293.0375, 107.8) centre (-293.5375, 107.8) ccw
  line L120 (-293.5375, 107.3) -> (-306.5375, 107.3)
  arc A101 (-307.0375, 107.8) -> (-306.5375, 107.3) centre (-306.5375, 107.8) ccw
  line L121 (-307.0375, 107.8) -> (-307.0375, 120.8)
  arc A102 (-306.5375, 121.3) -> (-307.0375, 120.8) centre (-306.5375, 120.8) ccw
  line L122 (-306.5375, 121.3) -> (-293.5375, 121.3)
  arc A103 (-293.0375, 120.8) -> (-293.5375, 121.3) centre (-293.5375, 120.8) ccw
  line L123 (-293.0375, 120.8) -> (-293.0375, 107.8)
  arc A104 (-169.7125, 69.2) -> (-169.2125, 69.7) centre (-169.7125, 69.7) ccw
  line L124 (-169.7125, 69.2) -> (-182.7125, 69.2)
  arc A105 (-183.2125, 69.7) -> (-182.7125, 69.2) centre (-182.7125, 69.7) ccw
  line L125 (-183.2125, 69.7) -> (-183.2125, 82.7)
  arc A106 (-182.7125, 83.2) -> (-183.2125, 82.7) centre (-182.7125, 82.7) ccw
  line L126 (-182.7125, 83.2) -> (-169.7125, 83.2)
  arc A107 (-169.2125, 82.7) -> (-169.7125, 83.2) centre (-169.7125, 82.7) ccw
  line L127 (-169.2125, 82.7) -> (-169.2125, 69.7)
  arc A108 (-29.2188, 107.3) -> (-28.7187, 107.8) centre (-29.2188, 107.8) ccw
  line L128 (-29.2188, 107.3) -> (-42.2188, 107.3)
  arc A109 (-42.7188, 107.8) -> (-42.2188, 107.3) centre (-42.2188, 107.8) ccw
  line L129 (-42.7188, 107.8) -> (-42.7188, 120.8)
  arc A110 (-42.2188, 121.3) -> (-42.7188, 120.8) centre (-42.2187, 120.8) ccw
  line L130 (-42.2188, 121.3) -> (-29.2188, 121.3)
  arc A111 (-28.7188, 120.8) -> (-29.2188, 121.3) centre (-29.2187, 120.8) ccw
  line L131 (-28.7188, 120.8) -> (-28.7187, 107.8)
  arc A112 (-60.175, 31.1) -> (-59.675, 31.6) centre (-60.175, 31.6) ccw
  line L132 (-60.175, 31.1) -> (-73.175, 31.1)
  arc A113 (-73.675, 31.6) -> (-73.175, 31.1) centre (-73.175, 31.6) ccw
  line L133 (-73.675, 31.6) -> (-73.675, 44.6)
  arc A114 (-73.175, 45.1) -> (-73.675, 44.6) centre (-73.175, 44.6) ccw
  line L134 (-73.175, 45.1) -> (-60.175, 45.1)
  arc A115 (-59.675, 44.6) -> (-60.175, 45.1) centre (-60.175, 44.6) ccw
  line L135 (-59.675, 44.6) -> (-59.675, 31.6)
  arc A116 (-312.5875, 107.3) -> (-312.0875, 107.8) centre (-312.5875, 107.8) ccw
  line L136 (-312.5875, 107.3) -> (-325.5875, 107.3)
  arc A117 (-326.0875, 107.8) -> (-325.5875, 107.3) centre (-325.5875, 107.8) ccw
  line L137 (-326.0875, 107.8) -> (-326.0875, 120.8)
  arc A118 (-325.5875, 121.3) -> (-326.0875, 120.8) centre (-325.5875, 120.8) ccw
  line L138 (-325.5875, 121.3) -> (-312.5875, 121.3)
  arc A119 (-312.0875, 120.8) -> (-312.5875, 121.3) centre (-312.5875, 120.8) ccw
  line L139 (-312.0875, 120.8) -> (-312.0875, 107.8)
  arc A120 (-126.85, 2.525) -> (-126.35, 3.025) centre (-126.85, 3.025) ccw
  line L140 (-126.85, 2.525) -> (-139.85, 2.525)
  arc A121 (-140.35, 3.025) -> (-139.85, 2.525) centre (-139.85, 3.025) ccw
  line L141 (-140.35, 3.025) -> (-140.35, 16.025)
  arc A122 (-139.85, 16.525) -> (-140.35, 16.025) centre (-139.85, 16.025) ccw
  line L142 (-139.85, 16.525) -> (-126.85, 16.525)
  arc A123 (-126.35, 16.025) -> (-126.85, 16.525) centre (-126.85, 16.025) ccw
  line L143 (-126.35, 16.025) -> (-126.35, 3.025)
  arc A124 (-331.6375, 2.525) -> (-331.1375, 3.025) centre (-331.6375, 3.025) ccw
  line L144 (-331.6375, 2.525) -> (-344.6375, 2.525)
  arc A125 (-345.1375, 3.025) -> (-344.6375, 2.525) centre (-344.6375, 3.025) ccw
  line L145 (-345.1375, 3.025) -> (-345.1375, 16.025)
  arc A126 (-344.6375, 16.525) -> (-345.1375, 16.025) centre (-344.6375, 16.025) ccw
  line L146 (-344.6375, 16.525) -> (-331.6375, 16.525)
  arc A127 (-331.1375, 16.025) -> (-331.6375, 16.525) centre (-331.6375, 16.025) ccw
  line L147 (-331.1375, 16.025) -> (-331.1375, 3.025)
  arc A128 (-164.95, 2.525) -> (-164.45, 3.025) centre (-164.95, 3.025) ccw
  line L148 (-164.95, 2.525) -> (-177.95, 2.525)
  arc A129 (-178.45, 3.025) -> (-177.95, 2.525) centre (-177.95, 3.025) ccw
  line L149 (-178.45, 3.025) -> (-178.45, 16.025)
  arc A130 (-177.95, 16.525) -> (-178.45, 16.025) centre (-177.95, 16.025) ccw
  line L150 (-177.95, 16.525) -> (-164.95, 16.525)
  arc A131 (-164.45, 16.025) -> (-164.95, 16.525) centre (-164.95, 16.025) ccw
  line L151 (-164.45, 16.025) -> (-164.45, 3.025)
  arc A132 (-184, 50.15) -> (-183.5, 50.65) centre (-184, 50.65) ccw
  line L152 (-184, 50.15) -> (-197, 50.15)
  arc A133 (-197.5, 50.65) -> (-197, 50.15) centre (-197, 50.65) ccw
  line L153 (-197.5, 50.65) -> (-197.5, 63.65)
  arc A134 (-197, 64.15) -> (-197.5, 63.65) centre (-197, 63.65) ccw
  line L154 (-197, 64.15) -> (-184, 64.15)
  arc A135 (-183.5, 63.65) -> (-184, 64.15) centre (-184, 63.65) ccw
  line L155 (-183.5, 63.65) -> (-183.5, 50.65)
  arc A136 (-331.6375, 31.1) -> (-331.1375, 31.6) centre (-331.6375, 31.6) ccw
  line L156 (-331.6375, 31.1) -> (-344.6375, 31.1)
  arc A137 (-345.1375, 31.6) -> (-344.6375, 31.1) centre (-344.6375, 31.6) ccw
  line L157 (-345.1375, 31.6) -> (-345.1375, 44.6)
  arc A138 (-344.6375, 45.1) -> (-345.1375, 44.6) centre (-344.6375, 44.6) ccw
  line L158 (-344.6375, 45.1) -> (-331.6375, 45.1)
  arc A139 (-331.1375, 44.6) -> (-331.6375, 45.1) centre (-331.6375, 44.6) ccw
  line L159 (-331.1375, 44.6) -> (-331.1375, 31.6)
  arc A140 (-155.425, 31.1) -> (-154.925, 31.6) centre (-155.425, 31.6) ccw
  line L160 (-155.425, 31.1) -> (-168.425, 31.1)
  arc A141 (-168.925, 31.6) -> (-168.425, 31.1) centre (-168.425, 31.6) ccw
  line L161 (-168.925, 31.6) -> (-168.925, 44.6)
  arc A142 (-168.425, 45.1) -> (-168.925, 44.6) centre (-168.425, 44.6) ccw
  line L162 (-168.425, 45.1) -> (-155.425, 45.1)
  arc A143 (-154.925, 44.6) -> (-155.425, 45.1) centre (-155.425, 44.6) ccw
  line L163 (-154.925, 44.6) -> (-154.925, 31.6)
  arc A144 (-126.85, 50.15) -> (-126.35, 50.65) centre (-126.85, 50.65) ccw
  line L164 (-126.85, 50.15) -> (-139.85, 50.15)
  arc A145 (-140.35, 50.65) -> (-139.85, 50.15) centre (-139.85, 50.65) ccw
  line L165 (-140.35, 50.65) -> (-140.35, 63.65)
  arc A146 (-139.85, 64.15) -> (-140.35, 63.65) centre (-139.85, 63.65) ccw
  line L166 (-139.85, 64.15) -> (-126.85, 64.15)
  arc A147 (-126.35, 63.65) -> (-126.85, 64.15) centre (-126.85, 63.65) ccw
  line L167 (-126.35, 63.65) -> (-126.35, 50.65)
  arc A148 (-195.9063, 107.3) -> (-195.4063, 107.8) centre (-195.9063, 107.8) ccw
  line L168 (-195.9063, 107.3) -> (-208.9062, 107.3)
  arc A149 (-209.4062, 107.8) -> (-208.9062, 107.3) centre (-208.9062, 107.8) ccw
  line L169 (-209.4062, 107.8) -> (-209.4062, 120.8)
  arc A150 (-208.9062, 121.3) -> (-209.4063, 120.8) centre (-208.9062, 120.8) ccw
  line L170 (-208.9062, 121.3) -> (-195.9063, 121.3)
  arc A151 (-195.4063, 120.8) -> (-195.9063, 121.3) centre (-195.9063, 120.8) ccw
  line L171 (-195.4063, 120.8) -> (-195.4063, 107.8)
  arc A152 (-212.575, 2.525) -> (-212.075, 3.025) centre (-212.575, 3.025) ccw
  line L172 (-212.575, 2.525) -> (-225.575, 2.525)
  arc A153 (-226.075, 3.025) -> (-225.575, 2.525) centre (-225.575, 3.025) ccw
  line L173 (-226.075, 3.025) -> (-226.075, 16.025)
  arc A154 (-225.575, 16.525) -> (-226.075, 16.025) centre (-225.575, 16.025) ccw
  line L174 (-225.575, 16.525) -> (-212.575, 16.525)
  arc A155 (-212.075, 16.025) -> (-212.575, 16.525) centre (-212.575, 16.025) ccw
  line L175 (-212.075, 16.025) -> (-212.075, 3.025)
  arc A156 (-3.025, 31.1) -> (-2.525, 31.6) centre (-3.025, 31.6) ccw
  line L176 (-3.025, 31.1) -> (-16.025, 31.1)
  arc A157 (-16.525, 31.6) -> (-16.025, 31.1) centre (-16.025, 31.6) ccw
  line L177 (-16.525, 31.6) -> (-16.525, 44.6)
  arc A158 (-16.025, 45.1) -> (-16.525, 44.6) centre (-16.025, 44.6) ccw
  line L178 (-16.025, 45.1) -> (-3.025, 45.1)
  arc A159 (-2.525, 44.6) -> (-3.025, 45.1) centre (-3.025, 44.6) ccw
  line L179 (-2.525, 44.6) -> (-2.525, 31.6)
  arc A160 (-243.5313, 107.3) -> (-243.0313, 107.8) centre (-243.5312, 107.8) ccw
  line L180 (-243.5313, 107.3) -> (-256.5313, 107.3)
  arc A161 (-257.0312, 107.8) -> (-256.5312, 107.3) centre (-256.5312, 107.8) ccw
  line L181 (-257.0312, 107.8) -> (-257.0313, 120.8)
  arc A162 (-256.5312, 121.3) -> (-257.0312, 120.8) centre (-256.5312, 120.8) ccw
  line L182 (-256.5312, 121.3) -> (-243.5312, 121.3)
  arc A163 (-243.0313, 120.8) -> (-243.5313, 121.3) centre (-243.5313, 120.8) ccw
  line L183 (-243.0312, 120.8) -> (-243.0312, 107.8)
  arc A164 (-212.575, 31.1) -> (-212.075, 31.6) centre (-212.575, 31.6) ccw
  line L184 (-212.575, 31.1) -> (-225.575, 31.1)
  arc A165 (-226.075, 31.6) -> (-225.575, 31.1) centre (-225.575, 31.6) ccw
  line L185 (-226.075, 31.6) -> (-226.075, 44.6)
  arc A166 (-225.575, 45.1) -> (-226.075, 44.6) centre (-225.575, 44.6) ccw
  line L186 (-225.575, 45.1) -> (-212.575, 45.1)
  arc A167 (-212.075, 44.6) -> (-212.575, 45.1) centre (-212.575, 44.6) ccw
  line L187 (-212.075, 44.6) -> (-212.075, 31.6)
  arc A168 (-141.1375, 88.25) -> (-140.6375, 88.75) centre (-141.1375, 88.75) ccw
  line L188 (-141.1375, 88.25) -> (-154.1375, 88.25)
  arc A169 (-154.6375, 88.75) -> (-154.1375, 88.25) centre (-154.1375, 88.75) ccw
  line L189 (-154.6375, 88.75) -> (-154.6375, 101.75)
  arc A170 (-154.1375, 102.25) -> (-154.6375, 101.75) centre (-154.1375, 101.75) ccw
  line L190 (-154.1375, 102.25) -> (-141.1375, 102.25)
  arc A171 (-140.6375, 101.75) -> (-141.1375, 102.25) centre (-141.1375, 101.75) ccw
  line L191 (-140.6375, 101.75) -> (-140.6375, 88.75)
  arc A172 (-5.4063, 107.3) -> (-4.9062, 107.8) centre (-5.4063, 107.8) ccw
  line L192 (-5.4062, 107.3) -> (-18.4062, 107.3)
  arc A173 (-18.9062, 107.8) -> (-18.4062, 107.3) centre (-18.4062, 107.8) ccw
  line L193 (-18.9062, 107.8) -> (-18.9062, 120.8)
  arc A174 (-18.4062, 121.3) -> (-18.9063, 120.8) centre (-18.4062, 120.8) ccw
  line L194 (-18.4062, 121.3) -> (-5.4062, 121.3)
  arc A175 (-4.9062, 120.8) -> (-5.4062, 121.3) centre (-5.4063, 120.8) ccw
  line L195 (-4.9062, 120.8) -> (-4.9062, 107.8)
  arc A176 (-79.225, 2.525) -> (-78.725, 3.025) centre (-79.225, 3.025) ccw
  line L196 (-79.225, 2.525) -> (-92.225, 2.525)
  arc A177 (-92.725, 3.025) -> (-92.225, 2.525) centre (-92.225, 3.025) ccw
  line L197 (-92.725, 3.025) -> (-92.725, 16.025)
  arc A178 (-92.225, 16.525) -> (-92.725, 16.025) centre (-92.225, 16.025) ccw
  line L198 (-92.225, 16.525) -> (-79.225, 16.525)
  arc A179 (-78.725, 16.025) -> (-79.225, 16.525) centre (-79.225, 16.025) ccw
  line L199 (-78.725, 16.025) -> (-78.725, 3.025)
  arc A180 (-184, 2.525) -> (-183.5, 3.025) centre (-184, 3.025) ccw
  line L200 (-184, 2.525) -> (-197, 2.525)
  arc A181 (-197.5, 3.025) -> (-197, 2.525) centre (-197, 3.025) ccw
  line L201 (-197.5, 3.025) -> (-197.5, 16.025)
  arc A182 (-197, 16.525) -> (-197.5, 16.025) centre (-197, 16.025) ccw
  line L202 (-197, 16.525) -> (-184, 16.525)
  arc A183 (-183.5, 16.025) -> (-184, 16.525) centre (-184, 16.025) ccw
  line L203 (-183.5, 16.025) -> (-183.5, 3.025)
  arc A184 (-193.525, 31.1) -> (-193.025, 31.6) centre (-193.525, 31.6) ccw
  line L204 (-193.525, 31.1) -> (-206.525, 31.1)
  arc A185 (-207.025, 31.6) -> (-206.525, 31.1) centre (-206.525, 31.6) ccw
  line L205 (-207.025, 31.6) -> (-207.025, 44.6)
  arc A186 (-206.525, 45.1) -> (-207.025, 44.6) centre (-206.525, 44.6) ccw
  line L206 (-206.525, 45.1) -> (-193.525, 45.1)
  arc A187 (-193.025, 44.6) -> (-193.525, 45.1) centre (-193.525, 44.6) ccw
  line L207 (-193.025, 44.6) -> (-193.025, 31.6)
  arc A188 (-41.125, 31.1) -> (-40.625, 31.6) centre (-41.125, 31.6) ccw
  line L208 (-41.125, 31.1) -> (-54.125, 31.1)
  arc A189 (-54.625, 31.6) -> (-54.125, 31.1) centre (-54.125, 31.6) ccw
  line L209 (-54.625, 31.6) -> (-54.625, 44.6)
  arc A190 (-54.125, 45.1) -> (-54.625, 44.6) centre (-54.125, 44.6) ccw
  line L210 (-54.125, 45.1) -> (-41.125, 45.1)
  arc A191 (-40.625, 44.6) -> (-41.125, 45.1) centre (-41.125, 44.6) ccw
  line L211 (-40.625, 44.6) -> (-40.625, 31.6)
  arc A192 (-269.725, 2.525) -> (-269.225, 3.025) centre (-269.725, 3.025) ccw
  line L212 (-269.725, 2.525) -> (-282.725, 2.525)
  arc A193 (-283.225, 3.025) -> (-282.725, 2.525) centre (-282.725, 3.025) ccw
  line L213 (-283.225, 3.025) -> (-283.225, 16.025)
  arc A194 (-282.725, 16.525) -> (-283.225, 16.025) centre (-282.725, 16.025) ccw
  line L214 (-282.725, 16.525) -> (-269.725, 16.525)
  arc A195 (-269.225, 16.025) -> (-269.725, 16.525) centre (-269.725, 16.025) ccw
  line L215 (-269.225, 16.025) -> (-269.225, 3.025)
  arc A196 (-293.5375, 88.25) -> (-293.0375, 88.75) centre (-293.5375, 88.75) ccw
  line L216 (-293.5375, 88.25) -> (-306.5375, 88.25)
  arc A197 (-307.0375, 88.75) -> (-306.5375, 88.25) centre (-306.5375, 88.75) ccw
  line L217 (-307.0375, 88.75) -> (-307.0375, 101.75)
  arc A198 (-306.5375, 102.25) -> (-307.0375, 101.75) centre (-306.5375, 101.75) ccw
  line L218 (-306.5375, 102.25) -> (-293.5375, 102.25)
  arc A199 (-293.0375, 101.75) -> (-293.5375, 102.25) centre (-293.5375, 101.75) ccw
  line L219 (-293.0375, 101.75) -> (-293.0375, 88.75)
  arc A200 (-331.6375, 107.3) -> (-331.1375, 107.8) centre (-331.6375, 107.8) ccw
  line L220 (-331.6375, 107.3) -> (-344.6375, 107.3)
  arc A201 (-345.1375, 107.8) -> (-344.6375, 107.3) centre (-344.6375, 107.8) ccw
  line L221 (-345.1375, 107.8) -> (-345.1375, 120.8)
  arc A202 (-344.6375, 121.3) -> (-345.1375, 120.8) centre (-344.6375, 120.8) ccw
  line L222 (-344.6375, 121.3) -> (-331.6375, 121.3)
  arc A203 (-331.1375, 120.8) -> (-331.6375, 121.3) centre (-331.6375, 120.8) ccw
  line L223 (-331.1375, 120.8) -> (-331.1375, 107.8)
  arc A204 (-64.9375, 88.25) -> (-64.4375, 88.75) centre (-64.9375, 88.75) ccw
  line L224 (-64.9375, 88.25) -> (-77.9375, 88.25)
  arc A205 (-78.4375, 88.75) -> (-77.9375, 88.25) centre (-77.9375, 88.75) ccw
  line L225 (-78.4375, 88.75) -> (-78.4375, 101.75)
  arc A206 (-77.9375, 102.25) -> (-78.4375, 101.75) centre (-77.9375, 101.75) ccw
  line L226 (-77.9375, 102.25) -> (-64.9375, 102.25)
  arc A207 (-64.4375, 101.75) -> (-64.9375, 102.25) centre (-64.9375, 101.75) ccw
  line L227 (-64.4375, 101.75) -> (-64.4375, 88.75)
  arc A208 (-188.7625, 69.2) -> (-188.2625, 69.7) centre (-188.7625, 69.7) ccw
  line L228 (-188.7625, 69.2) -> (-201.7625, 69.2)
  arc A209 (-202.2625, 69.7) -> (-201.7625, 69.2) centre (-201.7625, 69.7) ccw
  line L229 (-202.2625, 69.7) -> (-202.2625, 82.7)
  arc A210 (-201.7625, 83.2) -> (-202.2625, 82.7) centre (-201.7625, 82.7) ccw
  line L230 (-201.7625, 83.2) -> (-188.7625, 83.2)
  arc A211 (-188.2625, 82.7) -> (-188.7625, 83.2) centre (-188.7625, 82.7) ccw
  line L231 (-188.2625, 82.7) -> (-188.2625, 69.7)
  arc A212 (-98.275, 2.525) -> (-97.775, 3.025) centre (-98.275, 3.025) ccw
  line L232 (-98.275, 2.525) -> (-111.275, 2.525)
  arc A213 (-111.775, 3.025) -> (-111.275, 2.525) centre (-111.275, 3.025) ccw
  line L233 (-111.775, 3.025) -> (-111.775, 16.025)
  arc A214 (-111.275, 16.525) -> (-111.775, 16.025) centre (-111.275, 16.025) ccw
  line L234 (-111.275, 16.525) -> (-98.275, 16.525)
  arc A215 (-97.775, 16.025) -> (-98.275, 16.525) centre (-98.275, 16.025) ccw
  line L235 (-97.775, 16.025) -> (-97.775, 3.025)
  arc A216 (-331.6375, 69.2) -> (-331.1375, 69.7) centre (-331.6375, 69.7) ccw
  line L236 (-331.6375, 69.2) -> (-344.6375, 69.2)
  arc A217 (-345.1375, 69.7) -> (-344.6375, 69.2) centre (-344.6375, 69.7) ccw
  line L237 (-345.1375, 69.7) -> (-345.1375, 82.7)
  arc A218 (-344.6375, 83.2) -> (-345.1375, 82.7) centre (-344.6375, 82.7) ccw
  line L238 (-344.6375, 83.2) -> (-331.6375, 83.2)
  arc A219 (-331.1375, 82.7) -> (-331.6375, 83.2) centre (-331.6375, 82.7) ccw
  line L239 (-331.1375, 82.7) -> (-331.1375, 69.7)
  arc A220 (-131.6125, 69.2) -> (-131.1125, 69.7) centre (-131.6125, 69.7) ccw
  line L240 (-131.6125, 69.2) -> (-144.6125, 69.2)
  arc A221 (-145.1125, 69.7) -> (-144.6125, 69.2) centre (-144.6125, 69.7) ccw
  line L241 (-145.1125, 69.7) -> (-145.1125, 82.7)
  arc A222 (-144.6125, 83.2) -> (-145.1125, 82.7) centre (-144.6125, 82.7) ccw
  line L242 (-144.6125, 83.2) -> (-131.6125, 83.2)
  arc A223 (-131.1125, 82.7) -> (-131.6125, 83.2) centre (-131.6125, 82.7) ccw
  line L243 (-131.1125, 82.7) -> (-131.1125, 69.7)
  arc A224 (-79.225, 31.1) -> (-78.725, 31.6) centre (-79.225, 31.6) ccw
  line L244 (-79.225, 31.1) -> (-92.225, 31.1)
  arc A225 (-92.725, 31.6) -> (-92.225, 31.1) centre (-92.225, 31.6) ccw
  line L245 (-92.725, 31.6) -> (-92.725, 44.6)
  arc A226 (-92.225, 45.1) -> (-92.725, 44.6) centre (-92.225, 44.6) ccw
  line L246 (-92.225, 45.1) -> (-79.225, 45.1)
  arc A227 (-78.725, 44.6) -> (-79.225, 45.1) centre (-79.225, 44.6) ccw
  line L247 (-78.725, 44.6) -> (-78.725, 31.6)
  arc A228 (-231.625, 31.1) -> (-231.125, 31.6) centre (-231.625, 31.6) ccw
  line L248 (-231.625, 31.1) -> (-244.625, 31.1)
  arc A229 (-245.125, 31.6) -> (-244.625, 31.1) centre (-244.625, 31.6) ccw
  line L249 (-245.125, 31.6) -> (-245.125, 44.6)
  arc A230 (-244.625, 45.1) -> (-245.125, 44.6) centre (-244.625, 44.6) ccw
  line L250 (-244.625, 45.1) -> (-231.625, 45.1)
  arc A231 (-231.125, 44.6) -> (-231.625, 45.1) centre (-231.625, 44.6) ccw
  line L251 (-231.125, 44.6) -> (-231.125, 31.6)
  arc A232 (-22.075, 31.1) -> (-21.575, 31.6) centre (-22.075, 31.6) ccw
  line L252 (-22.075, 31.1) -> (-35.075, 31.1)
  arc A233 (-35.575, 31.6) -> (-35.075, 31.1) centre (-35.075, 31.6) ccw
  line L253 (-35.575, 31.6) -> (-35.575, 44.6)
  arc A234 (-35.075, 45.1) -> (-35.575, 44.6) centre (-35.075, 44.6) ccw
  line L254 (-35.075, 45.1) -> (-22.075, 45.1)
  arc A235 (-21.575, 44.6) -> (-22.075, 45.1) centre (-22.075, 44.6) ccw
  line L255 (-21.575, 44.6) -> (-21.575, 31.6)
  arc A236 (-74.4625, 69.2) -> (-73.9625, 69.7) centre (-74.4625, 69.7) ccw
  line L256 (-74.4625, 69.2) -> (-87.4625, 69.2)
  arc A237 (-87.9625, 69.7) -> (-87.4625, 69.2) centre (-87.4625, 69.7) ccw
  line L257 (-87.9625, 69.7) -> (-87.9625, 82.7)
  arc A238 (-87.4625, 83.2) -> (-87.9625, 82.7) centre (-87.4625, 82.7) ccw
  line L258 (-87.4625, 83.2) -> (-74.4625, 83.2)
  arc A239 (-73.9625, 82.7) -> (-74.4625, 83.2) centre (-74.4625, 82.7) ccw
  line L259 (-73.9625, 82.7) -> (-73.9625, 69.7)
  arc A240 (-217.3375, 88.25) -> (-216.8375, 88.75) centre (-217.3375, 88.75) ccw
  line L260 (-217.3375, 88.25) -> (-230.3375, 88.25)
  arc A241 (-230.8375, 88.75) -> (-230.3375, 88.25) centre (-230.3375, 88.75) ccw
  line L261 (-230.8375, 88.75) -> (-230.8375, 101.75)
  arc A242 (-230.3375, 102.25) -> (-230.8375, 101.75) centre (-230.3375, 101.75) ccw
  line L262 (-230.3375, 102.25) -> (-217.3375, 102.25)
  arc A243 (-216.8375, 101.75) -> (-217.3375, 102.25) centre (-217.3375, 101.75) ccw
  line L263 (-216.8375, 101.75) -> (-216.8375, 88.75)
  arc A244 (-145.9, 2.525) -> (-145.4, 3.025) centre (-145.9, 3.025) ccw
  line L264 (-145.9, 2.525) -> (-158.9, 2.525)
  arc A245 (-159.4, 3.025) -> (-158.9, 2.525) centre (-158.9, 3.025) ccw
  line L265 (-159.4, 3.025) -> (-159.4, 16.025)
  arc A246 (-158.9, 16.525) -> (-159.4, 16.025) centre (-158.9, 16.025) ccw
  line L266 (-158.9, 16.525) -> (-145.9, 16.525)
  arc A247 (-145.4, 16.025) -> (-145.9, 16.525) centre (-145.9, 16.025) ccw
  line L267 (-145.4, 16.025) -> (-145.4, 3.025)
  line L268 (-275.6852, 95.758) -> (-275.3216, 95.758)
  arc A248 (-275.3216, 95.758) -> (-274.8216, 96.258) centre (-275.3216, 96.258) ccw
  line L269 (-274.8216, 96.258) -> (-274.8216, 101.354)
  arc A249 (-274.3216, 101.854) -> (-274.8216, 101.354) centre (-274.3216, 101.354) ccw
  line L270 (-274.3216, 101.854) -> (-273.5183, 101.854)
  arc A250 (-273.5183, 101.854) -> (-273.0183, 102.354) centre (-273.5183, 102.354) ccw
  line L271 (-273.0183, 102.354) -> (-273.0183, 102.5224)
  arc A251 (-272.5183, 103.0224) -> (-273.0183, 102.5224) centre (-272.5183, 102.5224) ccw
  line L272 (-272.5183, 103.0224) -> (-270.4703, 103.0224)
  arc A252 (-269.9703, 102.5224) -> (-270.4703, 103.0224) centre (-270.4703, 102.5224) ccw
  line L273 (-269.9703, 102.5224) -> (-269.9703, 102.354)
  arc A253 (-269.9703, 102.354) -> (-269.4703, 101.854) centre (-269.4703, 102.354) ccw
  line L274 (-269.4703, 101.854) -> (-268.1669, 101.854)
  line L275 (-268.1669, 101.854) -> (-268.1669, 101.5666)
  arc A254 (-268.1669, 101.5666) -> (-267.6669, 101.0666) centre (-267.6669, 101.5666) ccw
  line L276 (-267.6669, 101.0666) -> (-266.5562, 101.0666)
  line L277 (-266.5562, 101.0666) -> (-266.5562, 101.75)
  arc A255 (-266.0562, 102.25) -> (-266.5562, 101.75) centre (-266.0563, 101.75) ccw
  line L278 (-266.0562, 102.25) -> (-253.0562, 102.25)
  arc A256 (-252.5562, 101.75) -> (-253.0562, 102.25) centre (-253.0562, 101.75) ccw
  line L279 (-252.5563, 101.75) -> (-252.5563, 101.0666)
  line L280 (-252.5563, 101.0666) -> (-251.4457, 101.0666)
  arc A257 (-251.4457, 101.0666) -> (-250.9457, 101.5666) centre (-251.4457, 101.5666) ccw
  line L281 (-250.9457, 101.5666) -> (-250.9457, 101.854)
  line L282 (-250.9457, 101.854) -> (-249.6422, 101.854)
  arc A258 (-249.6422, 101.854) -> (-249.1422, 102.354) centre (-249.6422, 102.354) ccw
  line L283 (-249.1423, 102.354) -> (-249.1423, 102.5224)
  arc A259 (-248.6423, 103.0224) -> (-249.1423, 102.5224) centre (-248.6423, 102.5224) ccw
  line L284 (-248.6423, 103.0224) -> (-246.5942, 103.0224)
  arc A260 (-246.0943, 102.5224) -> (-246.5942, 103.0224) centre (-246.5942, 102.5224) ccw
  line L285 (-246.0943, 102.5224) -> (-246.0943, 102.354)
  arc A261 (-246.0943, 102.354) -> (-245.5943, 101.854) centre (-245.5943, 102.354) ccw
  line L286 (-245.5943, 101.854) -> (-244.7909, 101.854)
  arc A262 (-244.2909, 101.354) -> (-244.7909, 101.854) centre (-244.7908, 101.354) ccw
  line L287 (-244.2909, 101.354) -> (-244.2909, 96.258)
  arc A263 (-244.2909, 96.258) -> (-243.7909, 95.758) centre (-243.7909, 96.258) ccw
  line L288 (-243.7909, 95.758) -> (-243.4273, 95.758)
  line L289 (-243.4273, 95.758) -> (-243.4272, 93.464)
  arc A264 (-243.9272, 92.964) -> (-243.4272, 93.464) centre (-243.9272, 93.464) ccw
  line L290 (-243.9272, 92.964) -> (-244.2909, 92.964)
  line L291 (-244.2909, 92.964) -> (-244.2909, 90.0604)
  arc A265 (-244.7909, 89.5604) -> (-244.2909, 90.0604) centre (-244.7909, 90.0604) ccw
  line L292 (-244.7909, 89.5604) -> (-250.4457, 89.5604)